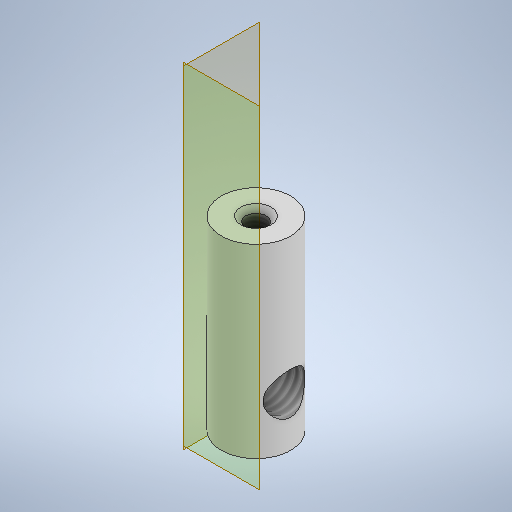
# Autodesk Inventor part: TS_V1_Fallmagazin_Zylinderanbindung_int
Saved by Autodesk Inventor 2025.2 (Build 292293000, 293)
## iProperties
Created: 2025-06-13
Part Number: TS_V1_Fallmagazin_Zylinderanbindung_int
Material: Generisch
Document SubType Name: Modeling
Designer: tino
Density: 1 g/cm^3
Appearance: Vorgabe
Author: tino
Autodesk Inventor part; units mm, degrees
ref_plane "XY Plane" through (0, 0, 0) normal (0, 0, 1) x (1, 0, 0)
sketch "Skizze1" plane through (0, 0, 0) normal (0, 0, 1) x (1, 0, 0)
  circle A0 centre (0, 0) radius 7
  dimension "d0" = 14
  constraints: 1 centre point, 1 coincident
  measures "d0" diameter of A0
extrude "Extrusion1" add sketch "Skizze1" along normal blind 37.5
sketch "Skizze2" plane through (0, 0, 37.5) normal (0, 0, 1) x (1, 0, 0)
  circle A0 centre (0, 0) radius 7 projected
hole "Bohrung1" at (0, 0, 37.5) direction (0, 0, -1) diameter 4.134 depth 12 tip angle 118 thread size "M5x0.8" class "6H" standard "ISO Metric profile"
chamfer "Fasen1" distance 1 angle 45 1 edges at (0, 2.067, 37.5)
ref_plane "Arbeitsebene1" through (-7, 0, 0) normal (1, 0, 0) x (0, 1, 0)
sketch "Skizze3" plane through (-7, 0, 0) normal (1, 0, 0) x (0, 1, 0)
  line L0 (7, 20) -> (-7, 20)
  line L1 (-7, 20) -> (-7, 0)
  line L2 (-7, 0) -> (7, 0)
  line L3 (7, 0) -> (7, 20)
  line L4 (7, 37.5) -> (-7, 37.5) projected
  line L5 (7, 0) -> (-7, 0) projected
  line L6 (7, 0) -> (7, 37.5) projected
  line L7 (-7, 0) -> (-7, 37.5) projected
  point P0 (0, 0)
  dimension "d13" = 20
  constraints: 8 end point, 3 collinear, 2 parallel, 1 horizontal, 1 perpendicular
  measures "d13" distance of L2.end L0.start
extrude "Extrusion2" cut sketch "Skizze3" along normal blind 2 contours L3 L2 L1 L0
sketch "Skizze4" plane through (-5, 0, 0) normal (-1, 0, 0) x (0, 0, 1)
  line L0 (0, -4.899) -> (0, 4.899) projected
  point P0 (0, 0)
  point P1 (10, 0)
  point P2 (0, 0)
  point P3 (0, 0)
  dimension "d17" = 10
  constraints: 2 midpoint, 1 horizontal alignment
  measures "d17" distance of point (0, 0) point (10, 0)
hole "Bohrung2" at (-5, 0, 10) direction (1, 0, 0) diameter 8.376 end through all thread size "M10x1.5" class "6H" standard "ISO Metric profile"
ref_plane "Arbeitsebene2" through (0, -7, 0) normal (0, 1, 0) x (-1, 0, 0)
sketch "Skizze5" plane through (0, -7, 0) normal (0, 1, 0) x (-1, 0, 0)
  line L0 (7, -7.5) -> (7, 45) projected
  line L1 (7, 20) -> (5, 20) projected
  line L2 (5, 20) -> (5, 0) projected
  line L3 (5, 20) -> (7, 22)
  line L4 (5, 20) -> (7.8284, 20) construction
  point P0 (0, 0)
  dimension "d25" = 45
  constraints: 4 end point, 1 equal length, 1 horizontal, 1 point on line
  measures "d25" angle of L4 L3
extrude "Extrusion3" cut sketch "Skizze5" along normal through all
